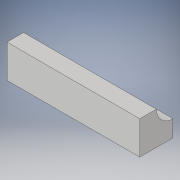
# Autodesk Inventor part: chuckFor_0_75_inchQuarterRound
Saved by Autodesk Inventor 2019.1 (Build 231200000, 200)
## iProperties
Created: 2018-09-04
Part Number: chuckFor_0_75_inchQuarterRound
Material: Generic
Document SubType Name: Modeling
Designer: steele
Density: 1 g/cm^3
Appearance: Default
Author: steele
Autodesk Inventor part; units mm, degrees
ref_plane "YZ Plane" through (0, 0, 0) normal (1, 0, 0) x (0, 1, 0)
ref_plane "XZ Plane" through (0, 0, 0) normal (0, 1, 0) x (-1, 0, 0)
ref_plane "XY Plane" through (0, 0, 0) normal (0, 0, 1) x (1, 0, 0)
sketch "Sketch1" plane through (0, 0, 0) normal (1, 0, 0) x (0, 1, 0)
  line L0 (0, 0) -> (38.1, 0)
  line L1 (38.1, 0) -> (38.1, -19.05)
  line L2 (19.05, -38.1) -> (0, -38.1)
  line L3 (0, -38.1) -> (0, 0)
  arc A0 (38.1, -19.05) -> (19.05, -38.1) centre (38.1, -38.1) ccw
  dimension "d0" = 38.1
  dimension "d1" = 38.1
  dimension "d2" = 38.1
  dimension "d5" = 38.1
  dimension "d6" = 38.1
  constraints: 8 end point, 2 parallel, 2 point on circle, 1 centre point, 1 horizontal, 1 perpendicular
  measures "d0" distance of L0.start L0.end
  measures "d1" distance of L2.end L0.start
  measures "d2" diameter of A0
  measures "d5" distance from line of A0.centre L3
  measures "d6" distance from line of L0 A0.centre
extrude "Extrusion1" add sketch "Sketch1" along normal mid plane 152.4
body "Solid1"
